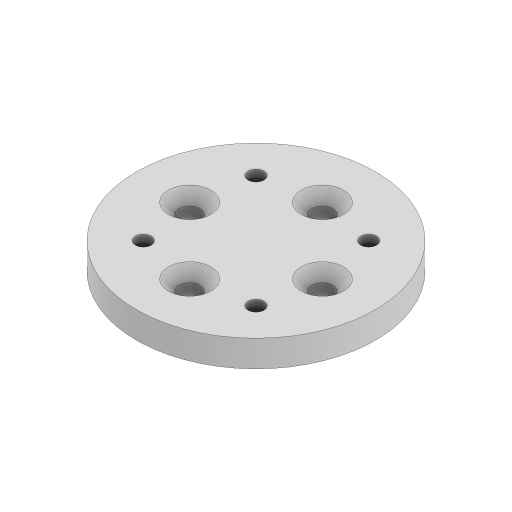
# Autodesk Inventor part: adaptador
Saved by Autodesk Inventor 2024.3 (Build 283343000, 343)
## iProperties
Created: 2025-03-05
Part Number: adaptador
Material: Generic
Document SubType Name: Modeling
Designer: danie
Density: 1 g/cm^3
Appearance: Default
Author: danie
Autodesk Inventor part; units mm, degrees
ref_plane "YZ Plane" through (0, 0, 0) normal (1, 0, 0) x (0, 1, 0)
ref_plane "XZ Plane" through (0, 0, 0) normal (0, 1, 0) x (-1, 0, 0)
ref_plane "XY Plane" through (0, 0, 0) normal (0, 0, 1) x (1, 0, 0)
sketch "Sketch1" plane through (0, 0, 0) normal (0, 1, 0) x (-1, 0, 0)
  circle A0 centre (0, 0) radius 12.5
  circle A1 centre (12.5, 0) radius 2
  circle A2 centre (0, 12.5) radius 2
  circle A3 centre (-12.5, 0) radius 2
  circle A4 centre (0, -12.5) radius 2
  circle A5 centre (0, 0) radius 22.5
  dimension "d0" = 25
  dimension "d1" = 4
  dimension "d4" = 360
  dimension "d6" = 45
  constraints: 5 centre point, 2 coincident, 1 horizontal alignment, 11 other
  measures "d1" diameter of A1
  measures "d6" diameter of A5
extrude "Extrusion1" add sketch "Sketch1" along normal blind 5 contours A1 A0 A4 A3 A2 | A5
chamfer "Chamfer1" distance 2 angle 45 4 edges at (-10.5, 5, 0) (2, 5, 12.5) (14.5, 5, 0) (2, 5, -12.5)
sketch "Sketch2" plane through (0, 5, 0) normal (0, 1, 0) x (1, 0, 0)
  circle A0 centre (0, 0) radius 15
  line L0 (0, 0) -> (-15, 0)
  line L1 (0, 0) -> (-10.6066, -10.6066)
  circle A1 centre (-10.6066, -10.6066) radius 1.5
  circle A2 centre (10.6066, -10.6066) radius 1.5
  circle A3 centre (10.6066, 10.6066) radius 1.5
  circle A4 centre (-10.6066, 10.6066) radius 1.5
  dimension "d12" = 30
  dimension "d13" = 45
  dimension "d14" = 3
  dimension "d17" = 360
  constraints: 5 centre point, 4 end point, 2 coincident, 2 point on circle, 1 horizontal, 9 other
  measures "d12" diameter of A0
  measures "d13" angle of L0 L1
  measures "d14" diameter of A1
extrude "Extrusion2" cut sketch "Sketch2" against normal blind 5 contours A3 A0 | A0 A3 | A2 A0 | A0 A2 | A4 A0 | A0 A4 | A1 A0 | A0 L1 A1 | A0 A1 L1
ref_plane "Work Plane1" through (0, 2.5, 0) normal (0, 1, 0) x (1, 0, 0)
sketch "Sketch4" plane through (0, 2.5, 0) normal (0, 1, 0) x (1, 0, 0)
  circle A0 centre (10.6066, 10.6066) radius 1.5 projected
  circle A1 centre (10.6066, -10.6066) radius 1.5 projected
  circle A2 centre (-10.6066, -10.6066) radius 1.5 projected
  circle A3 centre (-10.6066, 10.6066) radius 1.5 projected
  line L0 (13.3368, 8.9851) -> (10.5674, 7.4314)
  line L1 (10.5674, 7.4314) -> (7.8372, 9.0529)
  line L2 (7.8372, 9.0529) -> (7.8764, 12.2281)
  line L3 (7.8764, 12.2281) -> (10.6458, 13.7818)
  line L4 (10.6458, 13.7818) -> (13.376, 12.1603)
  line L5 (13.376, 12.1603) -> (13.3368, 8.9851)
  point P0 (0, 0)
  dimension "d28" = 5.5
  constraints: 12 end point, 1 coincident, 13 other
  measures "d28" distance between parallel lines of L3 L0
extrude "Extrusion3" cut sketch "Sketch4" along normal mid plane 2.2 contours L0 L1 L2 L3 L4 L5
pattern_circular "Circular Pattern1" count 4 over 360 about axis through (0, 0, 0) along (0, 1, 0) of "Extrusion3"
body "Solid1"
